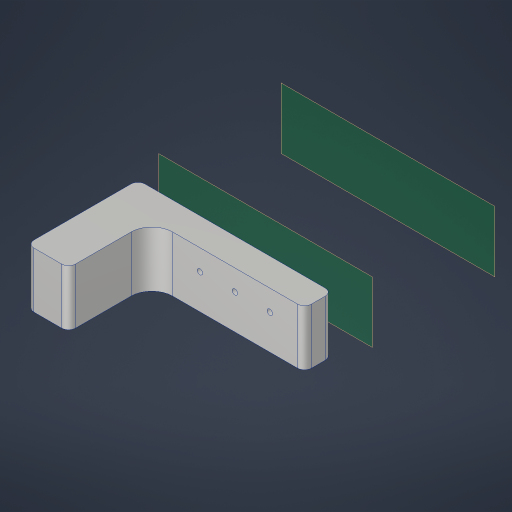
# Autodesk Inventor part: EL2-040
Saved by Autodesk Inventor 2023.4 (Build 274418000, 418)
## iProperties
Created: 2025-02-28
Part Number: EL2-040
Material: Aluminum 6061
Document SubType Name: Modeling
Designer: brand
Density: 2.7 g/cm^3
Appearance: Aluminum - Flat
Author: brand
Autodesk Inventor part; units mm, degrees
ref_plane "YZ Plane" through (0, 0, 0) normal (1, 0, 0) x (0, 1, 0)
ref_plane "XZ Plane" through (0, 0, 0) normal (0, 1, 0) x (-1, 0, 0)
ref_plane "XY Plane" through (0, 0, 0) normal (0, 0, 1) x (1, 0, 0)
sketch "Sketch1" plane through (0, 0, 0) normal (0, 0, 1) x (1, 0, 0)
  line L0 (-57.025, 9.525) -> (31.875, 9.525)
  line L1 (31.875, 9.525) -> (31.875, -15.875)
  line L2 (31.875, -15.875) -> (-57.025, -15.875)
  line L3 (-57.025, -15.875) -> (-57.025, 9.525)
  point P0 (0, 0)
  point P1 (16, 0)
  point P2 (-16, 0)
  point P3 (0, -8)
  dimension "d0" = 16
  dimension "d1" = 16
  dimension "d2" = 8
  dimension "d3" = 15.875
  dimension "d4" = 9.525
  dimension "d6" = 88.9
  dimension "d8" = 25.4
  constraints: 8 end point, 2 horizontal alignment, 2 parallel, 1 horizontal, 1 perpendicular, 1 vertical alignment
  measures "d0" distance of point (0, 0) point (-16, 0)
  measures "d1" distance of point (16, 0) point (0, 0)
  measures "d2" distance of point (0, 0) point (0, -8)
  measures "d3" distance from line of L1 point (16, 0)
  measures "d4" distance from line of L0 point (0, 0)
  measures "d6" distance between parallel lines of L3 L1
  measures "d8" distance of L2.end L0.start
extrude "Extrusion1" add sketch "Sketch1" along normal mid plane 50.8
sketch "Sketch2" plane through (-57.025, -15.875, -25.4) normal (-1, 0, 0) x (0, 0, -1)
  line L0 (-38.1635, -12.7) -> (-12.6365, -12.7) construction
  line L1 (0, -25.4) -> (-50.8, -25.4) construction
  line L2 (0, 0) -> (0, -25.4) construction
  point P0 (-25.4, -15.875)
  point P1 (-25.4, -12.7)
  point P2 (-25.4, -25.4)
  point P3 (0, -12.7)
  dimension "d18" = 25.527
  constraints: 2 end point, 2 midpoint, 1 horizontal, 1 horizontal alignment, 1 vertical alignment, 2 other
  measures "d18" distance of L0.start L0.end
hole "Hole2" at (-57.025, -3.175, -12.7635) at (-57.025, -3.175, 12.7635) direction (1, 0, 0) diameter 3.9624 depth 13.6144 thread size "10-32 UNF" class "2B" standard "ANSI Unified Screw Threads"
ref_plane "Work Plane2" through (0, 0, -39.3135) normal (0, 0, -1) x (-1, 0, 0)
ref_plane "Work Plane1" through (0, 0, -95.3135) normal (0, 0, -1) x (-1, 0, 0)
sketch "Sketch3" plane through (-57.025, 9.525, 25.4) normal (0, 1, 0) x (1, 0, 0)
  line L0 (0, 50.8) -> (0, 0) construction
  line L1 (88.9, 0) -> (0, 0) construction
  line L2 (88.9, 50.8) -> (88.9, 0) construction
  line L3 (0, 50.8) -> (88.9, 50.8) construction
  line L4 (88.9, 0) -> (0, 0) construction
  line L5 (9.525, 0) -> (9.525, 50.8) construction
  line L6 (0, 50.8) -> (88.9, 50.8) construction
  line L7 (0, 0) -> (88.9, 0) construction
  line L8 (88.9, 0) -> (19.05, 0)
  line L9 (19.05, 0) -> (19.05, 38.1)
  line L10 (19.05, 38.1) -> (88.9, 38.1)
  line L11 (88.9, 38.1) -> (88.9, 0)
  point P0 (57.025, 25.4)
  dimension "d28" = 9.525
  dimension "d29" = 12.7
  dimension "d30" = 19.05
  constraints: 10 end point, 2 parallel, 2 perpendicular, 2 point on line, 1 horizontal
  measures "d28" distance between parallel lines of L0 L5
  measures "d29" distance between parallel lines of L3 L10
  measures "d30" distance between parallel lines of L0 L9
extrude "Extrusion2" cut sketch "Sketch3" against normal through all
sketch "Sketch4" plane through (-37.975, 9.525, -12.7) normal (0, 0, 1) x (1, 0, 0)
  point P0 (37.975, -9.525)
  point P1 (21.975, -9.525)
  point P2 (37.975, -9.525)
  point P3 (53.975, -9.525)
hole "Hole3" at (-16, 0, -12.7) at (0, 0, -12.7) at (16, 0, -12.7) direction (0, 0, -1) diameter 2.459 depth 8.7884 thread size "M3x0.5" class "6H" standard "ANSI Metric M Profile"
fillet "Fillet1" radius 3.175 5 edges at (31.875, -3.175, -12.7) (31.875, -3.175, -25.4) (-37.975, -3.175, 25.4) (-57.025, -3.175, 25.4) (-57.025, -3.175, -25.4)
fillet "Fillet2" radius 9.525 1 edges at (-37.975, -3.175, -12.7)
equation "\"d1\" = d0"
body "Solid1"
